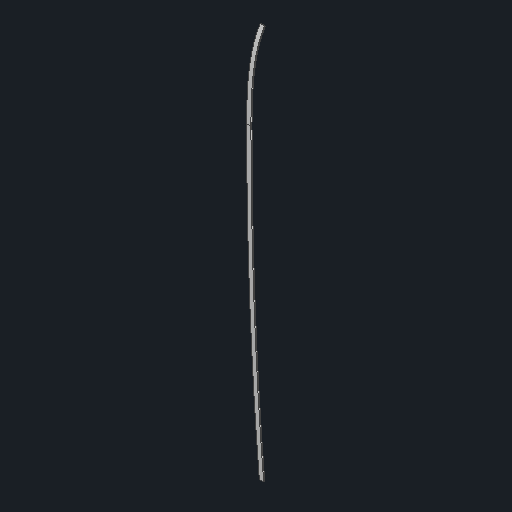
# Autodesk Inventor part: sealing_liner
Saved by Autodesk Inventor 2023 (Build 270158030, 158C)
## iProperties
Created: 2022-03-25
Part Number: sealing_liner
Material: Generic
Document SubType Name: Modeling
Designer: kardo
Density: 1 g/cm^3
Appearance: Default
Author: kardo
Autodesk Inventor part; units mm, degrees
ref_plane "YZ Plane" through (0, 0, 0) normal (1, 0, 0) x (0, 1, 0)
ref_plane "XZ Plane" through (0, 0, 0) normal (0, 1, 0) x (-1, 0, 0)
ref_plane "XY Plane" through (0, 0, 0) normal (0, 0, 1) x (1, 0, 0)
derived "parameters_frame.ipt"
derived "surface_body.ipt"
sketch "sk_rail_top_symmetry" plane through (0, 0, 0) normal (1, 0, 0) x (0, 1, 0)
  line L0 (0, 108.5007) -> (0, -224.6664) construction
  line L1 (0, 54.4) -> (-363, 54.4) construction
  line L2 (-363, 108.5007) -> (-363, -224.6664) construction
  line L3 (94.8, 108.5007) -> (94.8, -224.6664) construction
  line L4 (0, 54.4) -> (52.14, 54.4) construction
  line L5 (52.14, 54.4) -> (75.84, 49.3408) construction
  line L6 (75.84, 49.3408) -> (94.8, 37.536) construction
  line L7 (-487.5358, 0) -> (357.756, 0) construction
  spline S0 degree 2 poles (-363, 39.712) (-181.6483, 54.394) (0, 54.4) knots 0 0 0 1 1 1
  spline S1 degree 3 poles (0, 54.4) (52.14, 54.4) (75.84, 49.3408) (94.8, 37.536) knots 1 1 1 1 2 2 2 2
  point P0 (0, 0)
  point P1 (-181.5, 50.728)
  point P2 (94.8, 28.832)
ref_plane "plane_symmetry" through (0, 0, 0) normal (1, 0, 0) x (0, 1, 0)
sketch "sk_base" plane through (0, 0, 0) normal (1, 0, 0) x (0, 1, 0)
  spline S0 degree 2 poles (-363, 39.712) (-181.6483, 54.394) (0, 54.4) knots 0 0 0 1 1 1 projected
  spline S1 degree 3 poles (0, 54.4) (52.14, 54.4) (75.84, 49.3408) (94.8, 37.536) knots 1 1 1 1 2 2 2 2 projected
  line L0 (-362.9032, 38.5159) -> (-363, 39.712)
  line L1 (92.8, 38.7454) -> (92.1927, 37.7104)
  spline S2 degree 4 poles (-362.9032, 38.5159) (-272.3747, 45.845) (-181.6495, 50.7473) (-90.8247, 53.197) (0, 53.2) knots 0 0 0 0 0 1 1 1 1 1
  spline S3 degree 5 poles (0, 53.2) (8.694, 53.1996) (17.3891, 53.084) (26.0792, 52.8061) (40.7951, 51.9782) (55.4061, 50.0845) (61.3603, 49.0806) (71.3556, 46.8339) (80.9846, 43.3777) (84.8448, 41.7294) (88.5828, 39.8288) (92.1926, 37.7104) knots 0 0 0 0 0 0 0.459726 0.459726 0.459726 0.778684 0.778684 0.778684 1 1 1 1 1 1
  point P0 (0, 0)
  dimension "d7" = 1.2
  dimension "d8" = 2
  constraints: 4 end point, 9 other
  measures "d8" horizontal distance of point (94.8, 37.536) L1.start
extrude "thicken" add sketch "sk_base" along normal blind 5
equation "\"d7\" = cowl_liner_thickness"
equation "\"d8\" = bulkhead_thickness"
equation "\"d9\" = cowl_sealing_width"
equation "\"cowl_liner_thickness\" = 1.2"
equation "\"cowl_sealing_width\" = 5"
equation "\"bulkhead_thickness\" = 2"
body "Solid2"
